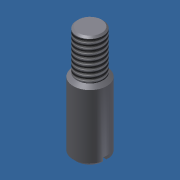
# Autodesk Inventor part: PINO ROSCADO(25)
Saved by Autodesk Inventor 2012 SP1 (Build 160190100, 190)
## iProperties
Created: 2012-07-24
Part Number: PINO ROSCADO(25)
Material: Carbon Steel
Document SubType Name: Modeling
Designer: bruno.silveira
Mass: 20.3976 g
Surface Area: 11.9381 cm^2
Volume: 2.59181 cm^3
Density: 7.87 g/cm^3
Author: bruno.silveira
Autodesk Inventor part; units mm, degrees
ref_plane "YZ Plane" through (0, 0, 0) normal (1, 0, 0) x (0, 1, 0)
ref_plane "XZ Plane" through (0, 0, 0) normal (0, 1, 0) x (-1, 0, 0)
ref_plane "XY Plane" through (0, 0, 0) normal (0, 0, 1) x (1, 0, 0)
sketch "Sketch1" plane through (0, 0, 0) normal (0, 0, 1) x (1, 0, 0)
  circle A0 centre (0, 0) radius 5
  dimension "d0" = 10
  constraints: 1 centre point, 1 coincident
  measures "d0" diameter of A0
extrude "Extrusion1" add sketch "Sketch1" along normal blind 33
sketch "Sketch2" plane through (0, 0, 33) normal (0, 0, 1) x (1, 0, 0)
  circle A0 centre (0, 0) radius 5 projected
  circle A1 centre (0, 0) radius 3.9688
  dimension "d3" = 7.9375
  constraints: 1 centre point, 1 coincident
  measures "d3" diameter of A1
extrude "Extrusion2" cut sketch "Sketch2" against normal blind 12
sketch "Sketch3" plane through (0, 0, 0) normal (0, 0, -1) x (-1, 0, 0)
  circle A0 centre (0, 0) radius 5 projected
  line L0 (-4.899, 1) -> (4.899, 1)
  line L1 (-4.899, -1) -> (4.899, -1)
  arc A1 (-4.899, 1) -> (-4.899, -1) centre (0, 0) ccw
  arc A2 (4.899, -1) -> (4.899, 1) centre (0, 0) ccw
  dimension "d6" = 2
  dimension "d8" = 1
  constraints: 8 point on circle, 4 end point, 2 centre point, 1 coincident
  measures "d6" distance between parallel lines of L0 L1
  measures "d8" distance from line of A0.centre L0
extrude "Extrusion3" cut sketch "Sketch3" against normal blind 2 contours A0 L1 L0
chamfer "Chamfer1" distance 1 angle 45 3 edges at (0, 5, 0) (0, -5, 0) (-5, 0, 21)
thread "Thread1" size "5/16-18 UNC" class "2A" standard "ANSI Unified Screw Threads" full length
chamfer "Chamfer2" distance 0.5 angle 45 1 edges at (-3.9688, 0, 33)
body "Solid1"
